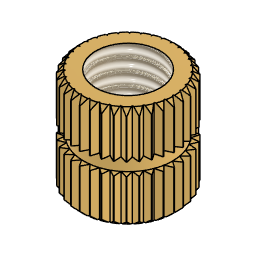
Insert M3x4x4 v1 (Autodesk Fusion 360 design; units mm, degrees)
Autodesk Fusion 360 part; units mm, degrees
note: some values were not read from the file. Set by a fixed rule: which sketch regions a step uses.
sketch "Sketch1" plane through (0, 0, 0) normal (0, 0, 1) x (1, 0, 0)
  circle A0 centre (0, 0) radius 2
  dimension "d1" = 4
  constraint coincident A0.centre origin
  measures "d1" diameter of A0
extrude "Extrude1" add sketch "Sketch1" along normal blind 4
chamfer "Chamfer1" distance 0.2 angle 45 2 edges at (-1.8647, -0.7232, 4) (-1.8647, -0.7232, 0)
sketch "Sketch2" plane through (0, 0, 0) normal (0, 0, 1) x (1, 0, 0)
  line L0 (0, 0) -> (2.1554, 0) construction
  circle A0 centre (0, 0) radius 1.75 construction
  line L1 (1.75, 0) -> (2.25, 0.3501)
  line L2 (2.25, 0.3501) -> (2.25, -0.3501)
  line L3 (2.25, -0.3501) -> (1.75, 0)
  dimension "d4" = 3.5
  dimension "d5" = 35
  dimension "d10" = 0.5
  constraint coincident L0.start A0.centre
  constraint horizontal L0
  constraint coincident A0 L1.start
  constraint coincident L0 L1.start
  constraint perpendicular L0 L2
  constraint symmetric L0 L1 L3
  measures "d4" diameter of A0
  measures "d5" angle of L0 L1
  measures "d10" distance of L1.start L2
extrude "Extrude2" cut sketch "Sketch2" along normal through all
pattern_circular "C-Pattern1" count 35 over 360 about axis through (0, 0, 0) along (0, 0, 1) of "Extrude2"
sketch "Sketch3" plane through (0, 0, 0) normal (0, 1, 0) x (1, 0, 0)
  line L0 (1.75, -2.25) -> (2.25, -2.25)
  line L1 (2.25, -2.25) -> (2.25, -1.75)
  line L2 (2.25, -1.75) -> (1.75, -1.75)
  line L3 (1.75, -1.75) -> (1.75, -2.25)
  line L4 (-2.4921, -2) -> (2.9857, -2) construction
  dimension "d11" = 2
  dimension "d12" = 0.5
  dimension "d13" = 1.75
  dimension "d14" = 0.5
  constraint horizontal L0
  constraint vertical L1
  constraint horizontal L2
  constraint vertical L3
  constraint perpendicular L1 L4
  constraint symmetric L0 L2 L4
  measures "d11" distance of origin L4
  measures "d12" distance of L0.end L1.end
  measures "d13" distance of origin L3
  measures "d14" distance of L0.start L0.end
revolve "Revolve1" cut sketch "Sketch3" angle 360 about axis through (0, 0, 1.75) along (0, 0, 1)
sketch "Sketch4" plane through (0, 0, 4) normal (0, 0, 1) x (-1, 0, 0)
  line L0 (-1.7219, 0.3125) -> (-1.777, 0.2871)
  arc A0 (-1.777, 0.2871) -> (-1.7997, 0.0348) centre (0, 0) ccw
  line L1 (-1.7997, 0.0348) -> (-1.75, 0)
  line L2 (-1.75, 0) -> (-1.7997, -0.0348)
  arc A1 (-1.7997, -0.0348) -> (-1.777, -0.2871) centre (0, 0) ccw
  line L3 (-1.777, -0.2871) -> (-1.7219, -0.3125)
  line L4 (-1.7219, -0.3125) -> (-1.7645, -0.3556)
  arc A2 (-1.7645, -0.3556) -> (-1.6971, -0.5998) centre (0, 0) ccw
  line L5 (-1.6971, -0.5998) -> (-1.6384, -0.6149)
  line L6 (-1.6384, -0.6149) -> (-1.6727, -0.6649)
  arc A3 (-1.6727, -0.6649) -> (-1.5628, -0.8932) centre (0, 0) ccw
  line L7 (-1.5628, -0.8932) -> (-1.5023, -0.8976)
  line L8 (-1.5023, -0.8976) -> (-1.5271, -0.9529)
  arc A4 (-1.5271, -0.9529) -> (-1.3782, -1.1579) centre (0, 0) ccw
  line L9 (-1.3782, -1.1579) -> (-1.3179, -1.1514)
  line L10 (-1.3179, -1.1514) -> (-1.3324, -1.2103)
  arc A5 (-1.3324, -1.2103) -> (-1.1493, -1.3854) centre (0, 0) ccw
  line L11 (-1.1493, -1.3854) -> (-1.0911, -1.3682)
  line L12 (-1.0911, -1.3682) -> (-1.0949, -1.4287)
  arc A6 (-1.0949, -1.4287) -> (-0.8834, -1.5683) centre (0, 0) ccw
  line L13 (-0.8834, -1.5683) -> (-0.8293, -1.541)
  line L14 (-0.8293, -1.541) -> (-0.8222, -1.6013)
  arc A7 (-0.8222, -1.6013) -> (-0.5892, -1.7008) centre (0, 0) ccw
  line L15 (-0.5892, -1.7008) -> (-0.5408, -1.6643)
  line L16 (-0.5408, -1.6643) -> (-0.5231, -1.7223)
  arc A8 (-0.5231, -1.7223) -> (-0.276, -1.7787) centre (0, 0) ccw
  line L17 (-0.276, -1.7787) -> (-0.2349, -1.7342)
  line L18 (-0.2349, -1.7342) -> (-0.2071, -1.788)
  arc A9 (-0.2071, -1.788) -> (0.046, -1.7994) centre (0, 0) ccw
  line L19 (0.046, -1.7994) -> (0.0785, -1.7482)
  line L20 (0.0785, -1.7482) -> (0.1155, -1.7963)
  arc A10 (0.1155, -1.7963) -> (0.3666, -1.7623) centre (0, 0) ccw
  line L21 (0.3666, -1.7623) -> (0.3894, -1.7061)
  line L22 (0.3894, -1.7061) -> (0.4344, -1.7468)
  arc A11 (0.4344, -1.7468) -> (0.6753, -1.6685) centre (0, 0) ccw
  line L23 (0.6753, -1.6685) -> (0.6878, -1.6092)
  line L24 (0.6878, -1.6092) -> (0.7393, -1.6412)
  arc A12 (0.7393, -1.6412) -> (0.9624, -1.5211) centre (0, 0) ccw
  line L25 (0.9624, -1.5211) -> (0.9641, -1.4605)
  line L26 (0.9641, -1.4605) -> (1.0205, -1.4828)
  arc A13 (1.0205, -1.4828) -> (1.2185, -1.3248) centre (0, 0) ccw
  line L27 (1.2185, -1.3248) -> (1.2094, -1.2649)
  line L28 (1.2094, -1.2649) -> (1.2688, -1.2768)
  arc A14 (1.2688, -1.2768) -> (1.4355, -1.0859) centre (0, 0) ccw
  line L29 (1.4355, -1.0859) -> (1.4158, -1.0286)
  line L30 (1.4158, -1.0286) -> (1.4764, -1.0297)
  arc A15 (1.4764, -1.0297) -> (1.6064, -0.8122) centre (0, 0) ccw
  line L31 (1.6064, -0.8122) -> (1.5767, -0.7593)
  line L32 (1.5767, -0.7593) -> (1.6365, -0.7495)
  arc A16 (1.6365, -0.7495) -> (1.7256, -0.5123) centre (0, 0) ccw
  line L33 (1.7256, -0.5123) -> (1.6869, -0.4656)
  line L34 (1.6869, -0.4656) -> (1.7441, -0.4453)
  arc A17 (1.7441, -0.4453) -> (1.7893, -0.196) centre (0, 0) ccw
  line L35 (1.7893, -0.196) -> (1.743, -0.1569)
  line L36 (1.743, -0.1569) -> (1.7955, -0.1267)
  arc A18 (1.7955, -0.1267) -> (1.7955, 0.1267) centre (0, 0) ccw
  line L37 (1.7955, 0.1267) -> (1.743, 0.1569)
  line L38 (1.743, 0.1569) -> (1.7893, 0.196)
  arc A19 (1.7893, 0.196) -> (1.7441, 0.4453) centre (0, 0) ccw
  line L39 (1.7441, 0.4453) -> (1.6869, 0.4656)
  line L40 (1.6869, 0.4656) -> (1.7256, 0.5123)
  arc A20 (1.7256, 0.5123) -> (1.6365, 0.7495) centre (0, 0) ccw
  line L41 (1.6365, 0.7495) -> (1.5767, 0.7593)
  line L42 (1.5767, 0.7593) -> (1.6064, 0.8122)
  arc A21 (1.6064, 0.8122) -> (1.4764, 1.0297) centre (0, 0) ccw
  line L43 (1.4764, 1.0297) -> (1.4158, 1.0286)
  line L44 (1.4158, 1.0286) -> (1.4355, 1.0859)
  arc A22 (1.4355, 1.0859) -> (1.2688, 1.2768) centre (0, 0) ccw
  line L45 (1.2688, 1.2768) -> (1.2094, 1.2649)
  line L46 (1.2094, 1.2649) -> (1.2185, 1.3248)
  arc A23 (1.2185, 1.3248) -> (1.0205, 1.4828) centre (0, 0) ccw
  line L47 (1.0205, 1.4828) -> (0.9641, 1.4605)
  line L48 (0.9641, 1.4605) -> (0.9624, 1.5211)
  arc A24 (0.9624, 1.5211) -> (0.7393, 1.6412) centre (0, 0) ccw
  line L49 (0.7393, 1.6412) -> (0.6878, 1.6092)
  line L50 (0.6878, 1.6092) -> (0.6753, 1.6685)
  arc A25 (0.6753, 1.6685) -> (0.4344, 1.7468) centre (0, 0) ccw
  line L51 (0.4344, 1.7468) -> (0.3894, 1.7061)
  line L52 (0.3894, 1.7061) -> (0.3666, 1.7623)
  arc A26 (0.3666, 1.7623) -> (0.1155, 1.7963) centre (0, 0) ccw
  line L53 (0.1155, 1.7963) -> (0.0785, 1.7482)
  line L54 (0.0785, 1.7482) -> (0.046, 1.7994)
  arc A27 (0.046, 1.7994) -> (-0.2071, 1.788) centre (0, 0) ccw
  line L55 (-0.2071, 1.788) -> (-0.2349, 1.7342)
  line L56 (-0.2349, 1.7342) -> (-0.276, 1.7787)
  arc A28 (-0.276, 1.7787) -> (-0.5231, 1.7223) centre (0, 0) ccw
  line L57 (-0.5231, 1.7223) -> (-0.5408, 1.6643)
  line L58 (-0.5408, 1.6643) -> (-0.5892, 1.7008)
  arc A29 (-0.5892, 1.7008) -> (-0.8222, 1.6013) centre (0, 0) ccw
  line L59 (-0.8222, 1.6013) -> (-0.8293, 1.541)
  line L60 (-0.8293, 1.541) -> (-0.8834, 1.5683)
  arc A30 (-0.8834, 1.5683) -> (-1.0949, 1.4287) centre (0, 0) ccw
  line L61 (-1.0949, 1.4287) -> (-1.0911, 1.3682)
  line L62 (-1.0911, 1.3682) -> (-1.1493, 1.3854)
  arc A31 (-1.1493, 1.3854) -> (-1.3324, 1.2103) centre (0, 0) ccw
  line L63 (-1.3324, 1.2103) -> (-1.3179, 1.1514)
  line L64 (-1.3179, 1.1514) -> (-1.3782, 1.1579)
  arc A32 (-1.3782, 1.1579) -> (-1.5271, 0.9529) centre (0, 0) ccw
  line L65 (-1.5271, 0.9529) -> (-1.5023, 0.8976)
  line L66 (-1.5023, 0.8976) -> (-1.5628, 0.8932)
  arc A33 (-1.5628, 0.8932) -> (-1.6727, 0.6649) centre (0, 0) ccw
  line L67 (-1.6727, 0.6649) -> (-1.6384, 0.6149)
  line L68 (-1.6384, 0.6149) -> (-1.6971, 0.5998)
  arc A34 (-1.6971, 0.5998) -> (-1.7645, 0.3556) centre (0, 0) ccw
  line L69 (-1.7645, 0.3556) -> (-1.7219, 0.3125)
  constraint coincident A0.centre A1.centre
hole "Hole1" at (0, 0, 4) direction (0, 0, -1) diameter 2.529 end through all
thread "Thread1" "ISO Metric profile 3.0 M3x0.5 6H" thread offset 0 thread depth 10
